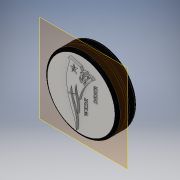
# Autodesk Inventor part: Wheel
Saved by Autodesk Inventor 2016 (Build 200138000, 138)
## iProperties
Created: 2016-10-07
Part Number: Wheel
Material: Generic
Document SubType Name: Modeling
Designer: desirw
Density: 1 g/cm^3
Appearance: Default
Mass: 52.9378 g
Surface Area: 147.304 cm^2
Volume: 52.9378 cm^3
Author: desirw
Autodesk Inventor part; units mm, degrees
ref_plane "YZ Plane" through (0, 0, 0) normal (1, 0, 0) x (0, 1, 0)
ref_plane "XZ Plane" through (0, 0, 0) normal (0, 1, 0) x (-1, 0, 0)
ref_plane "XY Plane" through (0, 0, 0) normal (0, 0, 1) x (1, 0, 0)
sketch "Sketch1" plane through (0, 0, 0) normal (0, 0, 1) x (1, 0, 0)
  circle A0 centre (0, 0) radius 31.75
  dimension "d0" = 63.5
  constraints: 1 centre point, 1 coincident
  measures "d0" diameter of A0
extrude "Extrusion1" add sketch "Sketch1" along normal blind 3.2512
sketch "Sketch2" plane through (0, 0, 3.2512) normal (0, 0, 1) x (1, 0, 0)
  circle A0 centre (0, 0) radius 33.655
  circle A1 centre (0, 0) radius 31.511
  circle A2 centre (0, 0) radius 31.511
  dimension "d3" = 67.31
  dimension "d40" = 2.144
  constraints: 3 centre point, 1 coincident
  measures "d3" diameter of A0
  measures "d40" radial gap between concentric circles of A1 A0
extrude "Extrusion2" add sketch "Sketch2" along normal blind 7.62 contours A0 | A1
sketch "Sketch3" plane through (0, 0, 0) normal (0, 0, -1) x (-1, 0, 0)
  circle A0 centre (0, 0) radius 33.655
  dimension "d6" = 67.31
  constraints: 1 centre point, 1 coincident
  measures "d6" diameter of A0
fillet "Fillet1" radius 2.54 1 edges at (-33.655, 0, 10.8712)
extrude "Extrusion3" add sketch "Sketch3" along normal blind 7.62
fillet "Fillet2" radius 2.54 1 edges at (33.655, 0, -7.62)
sketch "Sketch4" plane through (0, 0, -7.62) normal (0, 0, -1) x (-1, 0, 0)
  arc A0 (1.5256, -7.6067) -> (-1.5256, -7.6067) centre (0, -8.5367) ccw
  line L0 (1.5256, -7.6067) -> (10.0877, -14.0155)
  arc A1 (10.0877, -14.0155) -> (14.0155, -10.0877) centre (11.7691, -11.7691) ccw
  line L1 (14.0155, -10.0877) -> (7.6067, -1.5256)
  arc A2 (7.6067, 1.5256) -> (7.6067, -1.5256) centre (8.5367, 0) ccw
  line L2 (7.6067, 1.5256) -> (14.0155, 10.0877)
  arc A3 (14.0155, 10.0877) -> (10.0877, 14.0155) centre (11.7691, 11.7691) ccw
  line L3 (10.0877, 14.0155) -> (1.5256, 7.6067)
  arc A4 (-1.5256, 7.6067) -> (1.5256, 7.6067) centre (0, 8.5367) ccw
  line L4 (-1.5256, 7.6067) -> (-10.0877, 14.0155)
  arc A5 (-10.0877, 14.0155) -> (-14.0155, 10.0877) centre (-11.7691, 11.7691) ccw
  line L5 (-14.0155, 10.0877) -> (-7.6067, 1.5256)
  arc A6 (-7.6067, -1.5256) -> (-7.6067, 1.5256) centre (-8.5367, 0) ccw
  line L6 (-7.6067, -1.5256) -> (-14.0155, -10.0877)
  arc A7 (-14.0155, -10.0877) -> (-10.0877, -14.0155) centre (-11.7691, -11.7691) ccw
  line L7 (-10.0877, -14.0155) -> (-1.5256, -7.6067)
  circle A8 centre (12.339, -12.339) radius 0.75
  circle A9 centre (9.8641, -9.8641) radius 0.75
  circle A10 centre (7.3893, -7.3893) radius 0.75
  circle A11 centre (4.9144, -4.9144) radius 0.75
  circle A12 centre (12.339, 12.339) radius 0.75
  circle A13 centre (9.8641, 9.8641) radius 0.75
  circle A14 centre (7.3893, 7.3893) radius 0.75
  circle A15 centre (4.9144, 4.9144) radius 0.75
  circle A16 centre (-12.339, 12.339) radius 0.75
  circle A17 centre (-9.8641, 9.8641) radius 0.75
  circle A18 centre (-7.3893, 7.3893) radius 0.75
  circle A19 centre (-4.9144, 4.9144) radius 0.75
  circle A20 centre (-12.339, -12.339) radius 0.75
  circle A21 centre (-9.8641, -9.8641) radius 0.75
  circle A22 centre (-7.3893, -7.3893) radius 0.75
  circle A23 centre (-4.9144, -4.9144) radius 0.75
  circle A24 centre (0, 0) radius 3.6
  constraints: 25 centre point, 16 end point, 16 point on circle
extrude "Extrusion4" cut sketch "Sketch4" against normal blind 2.3622 contours A0 L7 A7 L6 A6 L5 A5 L4 A4 L3 A3 L2 A2 L1 A1 L0 | A8 | A9 | A10 | A11 | A12 | A13 | A14 | A15 | A16 | A17 | A18 | A19 | A20 | A21 | A22 | A23 | A24
sketch "Sketch5" plane through (0, 0, -7.62) normal (0, 0, -1) x (-1, 0, 0)
  circle A0 centre (0, 0) radius 3.6195
  dimension "d15" = 7.239
  constraints: 1 centre point, 1 coincident
  measures "d15" diameter of A0
extrude "Extrusion5" cut sketch "Sketch5" against normal blind 1.1684
sketch "Sketch6" plane through (0, 0, -5.2578) normal (0, 0, -1) x (-1, 0, 0)
  circle A0 centre (0, 0) radius 1.2446
  dimension "d16" = 2.4892
  constraints: 1 centre point, 1 coincident
  measures "d16" diameter of A0
extrude "Extrusion6" cut sketch "Sketch6" against normal blind 7.62
sketch "Sketch7" plane through (0, 0, 10.8712) normal (0, 0, 1) x (1, 0, 0)
  circle A0 centre (0, 0) radius 2.54
  dimension "d19" = 5.08
  constraints: 1 centre point, 1 coincident
  measures "d19" diameter of A0
extrude "Extrusion7" cut sketch "Sketch7" against normal blind 15.24
sketch "Sketch12" plane through (0, 0, -5.2578) normal (0, 0, -1) x (-1, 0, 0)
  circle A0 centre (0, 0) radius 3.5498
  circle A1 centre (0, 0) radius 3.6 projected
  dimension "d41" = 7.2
  constraints: 1 centre point, 1 coincident
  measures "d41" diameter of A1
extrude "Extrusion11" cut sketch "Sketch12" against normal blind 0.2286 contours A0
sketch "Sketch13" plane through (0, 0, -7.62) normal (0, 0, -1) x (-1, 0, 0)
  circle A0 centre (-9.8641, -9.8641) radius 1.0795
  circle A1 centre (-9.8641, 9.8641) radius 1.0795
  circle A2 centre (9.8641, 9.8641) radius 1.0795
  circle A3 centre (9.8641, -9.8641) radius 1.0795
  dimension "d46" = 2.159
  dimension "d48" = 2.159
  dimension "d49" = 2.159
  dimension "d50" = 2.159
  constraints: 4 centre point
  measures "d46" diameter of A0
  measures "d48" diameter of A2
  measures "d49" diameter of A3
  measures "d50" diameter of A1
extrude "Extrusion12" cut sketch "Sketch13" against normal blind 12.7
sketch "Sketch16" plane through (0, 0, 10.8712) normal (0, 0, 1) x (1, 0, 0)
  circle A0 centre (0, 0) radius 31.115 projected
  circle A1 centre (0, 0) radius 2.54 projected
  circle A2 centre (0, 0) radius 31.115
  constraints: 1 centre point, 1 coincident, 1 concentric
extrude "Extrusion13" cut sketch "Sketch16" against normal blind 2.54
sketch "Sketch17" plane through (0, 0, 8.3312) normal (0, 0, 1) x (1, 0, 0)
  circle A0 centre (0, 0) radius 1.2446 projected
  circle A1 centre (0, 0) radius 7.62
  circle A2 centre (0, 0) radius 29.21
  dimension "d56" = 15.24
  dimension "d60" = 58.42
  constraints: 2 centre point, 2 coincident
  measures "d56" diameter of A1
  measures "d60" diameter of A2
extrude "Extrusion14" cut sketch "Sketch17" against normal blind 12.7 contours A2
fillet "Fillet3" radius 3.175 2 edges at (-29.21, 0, 8.3312) (-7.62, 0, 8.3312)
sketch "Sketch20" plane through (0, 0, -7.62) normal (0, 0, -1) x (-1, 0, 0)
  circle A0 centre (19.0012, 0) radius 8.4433
  circle A1 centre (0, 0) radius 1.2446 projected
  circle A2 centre (0, 0) radius 2.54 projected
  circle A3 centre (0, -19.0012) radius 8.4433
  circle A4 centre (-19.0012, 0) radius 8.4433
  circle A5 centre (0, 19.0012) radius 8.4433
  arc A6 (15.9108, 14.6269) -> (13.5038, 17.0339) centre (16.1061, 17.2292) ccw construction
  arc A7 (15.8105, 13.2894) -> (12.1662, 16.9336) centre (16.1061, 17.2292) ccw
  arc A8 (16.0112, 15.9644) -> (14.8413, 17.1343) centre (16.1061, 17.2292) ccw
  arc A9 (16.0112, 15.9644) -> (15.8105, 13.2894) centre (15.9108, 14.6269) ccw
  arc A10 (12.1662, 16.9336) -> (14.8413, 17.1343) centre (13.5038, 17.0339) ccw
  arc A11 (14.6269, -15.9108) -> (17.0339, -13.5038) centre (17.2292, -16.1061) ccw construction
  arc A12 (13.2894, -15.8105) -> (16.9336, -12.1662) centre (17.2292, -16.1061) ccw
  arc A13 (15.9644, -16.0112) -> (17.1343, -14.8413) centre (17.2292, -16.1061) ccw
  arc A14 (15.9644, -16.0112) -> (13.2894, -15.8105) centre (14.6269, -15.9108) ccw
  arc A15 (16.9336, -12.1662) -> (17.1343, -14.8413) centre (17.0339, -13.5038) ccw
  arc A16 (-15.9108, -14.6269) -> (-13.5038, -17.0339) centre (-16.1061, -17.2292) ccw construction
  arc A17 (-15.8105, -13.2894) -> (-12.1662, -16.9336) centre (-16.1061, -17.2292) ccw
  arc A18 (-16.0112, -15.9644) -> (-14.8413, -17.1343) centre (-16.1061, -17.2292) ccw
  arc A19 (-16.0112, -15.9644) -> (-15.8105, -13.2894) centre (-15.9108, -14.6269) ccw
  arc A20 (-12.1662, -16.9336) -> (-14.8413, -17.1343) centre (-13.5038, -17.0339) ccw
  arc A21 (-14.6269, 15.9108) -> (-17.0339, 13.5038) centre (-17.2292, 16.1061) ccw construction
  arc A22 (-13.2894, 15.8105) -> (-16.9336, 12.1662) centre (-17.2292, 16.1061) ccw
  arc A23 (-15.9644, 16.0112) -> (-17.1343, 14.8413) centre (-17.2292, 16.1061) ccw
  arc A24 (-15.9644, 16.0112) -> (-13.2894, 15.8105) centre (-14.6269, 15.9108) ccw
  arc A25 (-16.9336, 12.1662) -> (-17.1343, 14.8413) centre (-17.0339, 13.5038) ccw
  dimension "d66" = 360
  dimension "d70" = 360
  constraints: 40 point on circle, 24 centre point, 4 coincident, 4 tangent, 67 other
extrude "Extrusion15" cut sketch "Sketch20" against normal blind 10.16 contours A0 | A3 | A4 | A5 | A9 A8 A10 A7 | A14 A13 A15 A12 | A19 A18 A20 A17 | A24 A23 A25 A22
sketch "Sketch21" plane through (0, 0, -4.3688) normal (0, 0, 1) x (1, 0, 0)
  circle A0 centre (-9.8653, -9.893) radius 2.159
  circle A1 centre (-9.8653, 9.8376) radius 2.159
  circle A2 centre (9.867, -9.893) radius 2.159
  circle A3 centre (9.867, 9.8376) radius 2.159
  point P0 (0, 0)
  dimension "d74" = 4.318
  dimension "d75" = 4.318
  dimension "d76" = 4.318
  dimension "d77" = 4.318
  constraints: 4 centre point
  measures "d74" diameter of A0
  measures "d75" diameter of A1
  measures "d76" diameter of A2
  measures "d77" diameter of A3
extrude "Extrusion16" cut sketch "Sketch21" against normal blind 0.254
sketch "Sketch23" plane through (0, 0, 8.3312) normal (0, 0, 1) x (1, 0, 0)
  circle A0 centre (0, 0) radius 8.0486
  constraints: 1 centre point, 1 coincident
extrude "Extrusion17" cut sketch "Sketch23" against normal blind 12.7
ref_plane "Work Plane2" through (0, 0, 8.3312) normal (0, 0, 1) x (1, 0, 0)
sketch "Sketch24" plane through (0, 0, 8.3312) normal (0, 0, 1) x (1, 0, 0)
  circle A0 centre (0, 0) radius 31.1534
  constraints: 1 centre point, 1 coincident
extrude "Extrusion18" add sketch "Sketch24" along normal blind 2.54
sketch "Sketch25" plane through (0, 0, 10.8712) normal (0, 0, 1) x (1, 0, 0)
  line L0 (-12.7986, -29.9392) -> (-12.7986, 28.2876) construction
  line L1 (-12.7986, 28.2876) -> (14.4515, 28.2876) construction
  line L2 (14.4515, 28.2876) -> (14.4515, -29.9392) construction
  line L3 (14.4515, -29.9392) -> (-12.7986, -29.9392) construction
  arc A0 (-2.4703, -28.2892) -> (-5.6682, -15.7345) centre (-39.8581, -31.1279) ccw
  arc A1 (-10.3026, -1.9948) -> (-5.6682, -15.7345) centre (146.9864, 43.407) ccw
  arc A2 (-2.4703, -28.2892) -> (-2.4703, -18.2629) centre (-33.8456, -23.2761) ccw
  arc A3 (-2.4703, -18.2629) -> (-5.2168, -8.4433) centre (-79.7357, -34.5801) ccw
  arc A4 (-7.0459, -1.252) -> (-5.2168, -8.4433) centre (32.2007, 4.9019) ccw
  line L4 (-10.3026, -1.9948) -> (-7.0459, -1.252)
  arc A5 (-1.4091, -14.8666) -> (-3.8781, -5.8135) centre (-42.9348, -21.3286) ccw
  arc A6 (-5.6682, -0.6984) -> (-3.8781, -5.8135) centre (38.7717, 11.9828) ccw
  arc A7 (-2.9605, 0) -> (-5.6682, -0.6984) centre (0.5008, -19.0171) ccw
  arc A8 (-1.7257, -5.5998) -> (-2.9605, 0) centre (-46.1597, -12.462) ccw
  arc A9 (-1.4091, -14.8666) -> (-1.7257, -5.5998) centre (-31.0492, -11.2405) ccw
  arc A10 (13.0542, 18.6707) -> (0.223, -3.0699) centre (34.2938, -8.5214) ccw
  arc A11 (13.0542, 18.6707) -> (11.4718, 20.2531) centre (10.1474, 17.3464) ccw
  arc A12 (11.4718, 20.2531) -> (9.4266, 20.0581) centre (10.5991, 18.5838) ccw
  arc A13 (9.4266, 20.0581) -> (8.2975, 20.459) centre (7.7468, 17.1172) ccw
  arc A14 (8.2975, 20.459) -> (7.2209, 20.5419) centre (7.4283, 16.2053) ccw
  arc A15 (6.4262, 22.0118) -> (7.2209, 20.5419) centre (11.9084, 24.0263) ccw
  arc A16 (2.6562, 21.2483) -> (6.4262, 22.0118) centre (-20.9306, 147.4079) ccw
  arc A17 (2.6562, 21.2483) -> (1.1935, 24.0263) centre (-252.5291, -111.3406) ccw
  arc A18 (1.1935, 24.0263) -> (-9.4849, 27.0616) centre (-900.7825, -3128.8756) ccw
  arc A19 (-9.1238, 22.0118) -> (-9.4849, 27.0616) centre (-21.4008, 23.6716) ccw
  arc A20 (-10.3026, 17.8312) -> (-9.1238, 22.0118) centre (-36.152, 27.3765) ccw
  arc A21 (-10.3026, 17.8312) -> (-11.3285, 12.6153) centre (170.6673, -20.4736) ccw
  arc A22 (-11.3285, 12.6153) -> (-10.3026, -1.252) centre (38.6762, 9.3432) ccw
  arc A23 (-7.374, -0.5894) -> (-10.3026, -1.252) centre (0.434, -41.9034) ccw
  arc A24 (-6.6405, 5.393) -> (-7.374, -0.5894) centre (2.9307, 1.1832) ccw
  arc A25 (-6.6405, 5.393) -> (-5.8275, -0.1263) centre (42.4689, 9.8072) ccw
  arc A26 (-3.1357, 0.5919) -> (-5.8275, -0.1263) centre (0.6817, -19.118) ccw
  arc A27 (-2.2091, 8.7203) -> (-3.1357, 0.5919) centre (7.8506, 3.4565) ccw
  arc A28 (-2.2091, 8.7203) -> (-1.4091, 2.4558) centre (41.2883, 11.0914) ccw
  arc A29 (0.223, -3.0699) -> (-1.4091, 2.4558) centre (-65.3016, -19.4203) ccw
  arc A30 (6.7707, 15.7398) -> (4.847, 15.3673) centre (16.1173, -37.684) ccw
  arc A31 (4.847, 15.3673) -> (2.5284, 11.9828) centre (51.1574, -18.8455) ccw
  arc A32 (2.0647, 12.0311) -> (2.5284, 11.9828) centre (2.3182, 12.2154) ccw
  arc A33 (0.6817, 14.3084) -> (2.0647, 12.0311) centre (3.8781, 14.6909) ccw
  arc A34 (1.0059, 16.9464) -> (0.6817, 14.3084) centre (8.9448, 14.6319) ccw
  arc A35 (1.507, 17.4809) -> (1.0059, 16.9464) centre (1.5569, 16.9319) ccw
  arc A36 (1.507, 17.4809) -> (1.791, 15.7398) centre (3.5637, 16.9227) ccw
  arc A37 (1.791, 15.7398) -> (2.9878, 14.8708) centre (3.5637, 16.9227) ccw
  line L5 (2.9878, 14.8708) -> (2.9878, 18.3662)
  arc A38 (1.4604, 19.4854) -> (2.9878, 18.3662) centre (3.1078, 20.1318) ccw
  arc A39 (1.3568, 19.6561) -> (1.4604, 19.4854) centre (1.5862, 19.6786) ccw
  arc A40 (1.3568, 20.1992) -> (1.3568, 19.6561) centre (2.2724, 19.9277) ccw
  arc A41 (5.9606, 21.1505) -> (1.3568, 20.1992) centre (8.9783, -5.0691) ccw
  line L6 (5.9606, 21.1505) -> (5.9606, 18.988)
  arc A42 (5.9606, 18.988) -> (6.2957, 18.7748) centre (9.575, 24.2979) ccw
  arc A43 (6.2957, 18.7748) -> (6.9567, 19.9277) centre (-103.158, 82.2966) ccw
  arc A44 (7.5209, 19.9277) -> (6.9567, 19.9277) centre (7.2388, 19.3131) ccw
  line L7 (7.5209, 19.9277) -> (7.5209, 18.6986)
  arc A45 (8.344, 17.7097) -> (7.5209, 18.6986) centre (6.084, 16.6658) ccw
  arc A46 (8.344, 17.7097) -> (8.1842, 18.8788) centre (6.4633, 18.0481) ccw
  line L8 (8.1842, 18.8788) -> (8.1842, 20.0692)
  line L9 (8.1842, 20.0692) -> (8.4773, 20.0692)
  arc A47 (9.1501, 19.6561) -> (8.4773, 20.0692) centre (8.1291, 18.7477) ccw
  line L10 (9.1501, 19.6561) -> (9.1501, 18.878)
  arc A48 (10.3252, 19.7825) -> (9.1501, 18.878) centre (11.157, 17.4862) ccw
  line L11 (10.3252, 19.7825) -> (10.9883, 19.7825)
  arc A49 (12.0805, 18.8788) -> (10.9883, 19.7825) centre (10.1284, 17.6314) ccw
  arc A50 (12.0805, 18.8788) -> (5.0259, 10.9955) centre (36.9587, -10.4824) ccw
  arc A51 (4.3066, 11.9036) -> (5.0259, 10.9955) centre (5.7027, 12.2705) ccw
  arc A52 (4.3066, 12.6373) -> (4.3066, 11.9036) centre (5.7027, 12.2705) ccw
  arc A53 (6.7707, 15.7398) -> (4.3066, 12.6373) centre (9.0478, 11.4015) ccw
  line L12 (-3.2282, 19.8186) -> (-2.0723, 16.5796)
  line L13 (-2.0723, 16.5796) -> (-4.5876, 18.4941)
  line L14 (-4.5876, 18.4941) -> (-6.5126, 16.6185)
  line L15 (-6.5126, 16.6185) -> (-5.8751, 19.474)
  line L16 (-5.8751, 19.474) -> (-7.5613, 20.8788)
  line L17 (-7.5613, 20.8788) -> (-5.366, 21.4271)
  line L18 (-5.366, 21.4271) -> (-4.6252, 24.0672)
  line L19 (-4.6252, 24.0672) -> (-3.8073, 21.7551)
  line L20 (-3.8073, 21.7551) -> (-0.8504, 22.1353)
  line L21 (-0.8504, 22.1353) -> (-3.2282, 19.8186)
  point P0 (0, 0)
  constraints: 110 point on circle, 54 centre point, 36 end point, 5 vertical, 3 concentric, 2 point on line, 1 collinear, 1 horizontal, 1 perpendicular, 2 other
extrude "Extrusion19" add sketch "Sketch25" along normal blind 2.032
sketch "Sketch26" plane through (0, 0, 10.8712) normal (0, 0, 1) x (1, 0, 0)
  line L0 (3.1838, -14.6945) -> (3.1838, -9.0616) construction
  line L1 (3.1838, -9.0616) -> (14.0414, -9.0616) construction
  line L2 (14.0414, -9.0616) -> (14.0414, -14.6945) construction
  line L3 (14.0414, -14.6945) -> (3.1838, -14.6945) construction
  line L4 (11.7993, -0.1306) -> (11.8156, 13.1695) construction
  line L5 (11.8156, 13.1695) -> (15.003, 13.1656) construction
  line L6 (15.003, 13.1656) -> (14.9868, -0.1345) construction
  line L7 (14.9868, -0.1345) -> (11.7993, -0.1306) construction
  line L8 (3.1838, -9.945) -> (3.2694, -9.945)
  spline S0 degree 2 poles (3.2694, -9.945) (3.2772, -10.0332) (3.3602, -10.1551) (3.4484, -10.2018) knots 0 0 0 1 2 2 2
  spline S1 degree 2 poles (3.4484, -10.2018) (3.4769, -10.2148) (3.8116, -10.3471) knots 0 0 0 1 1 1
  line L9 (3.8116, -10.3471) -> (6.4314, -11.3431)
  line L10 (6.4314, -11.3431) -> (6.4314, -11.4339)
  line L11 (6.4314, -11.4339) -> (4.3744, -12.2199)
  line L12 (4.3744, -12.2199) -> (6.4314, -13.0863)
  line L13 (6.4314, -13.0863) -> (6.4314, -13.1719)
  line L14 (6.4314, -13.1719) -> (3.8375, -14.2172)
  spline S2 degree 2 poles (3.8375, -14.2172) (3.4484, -14.3755) (3.2824, -14.5026) (3.2694, -14.653) knots 0 0 0 1 2 2 2
  line L15 (3.2694, -14.653) -> (3.1838, -14.653)
  line L16 (3.1838, -14.653) -> (3.1838, -13.2782)
  line L17 (3.1838, -13.2782) -> (3.2694, -13.2782)
  spline S3 degree 2 poles (3.2694, -13.2782) (3.2746, -13.4442) (3.3654, -13.5532) (3.4328, -13.5532) knots 0 0 0 1 2 2 2
  spline S4 degree 2 poles (3.4328, -13.5532) (3.5236, -13.5532) (3.8116, -13.4391) knots 0 0 0 1 1 1
  line L18 (3.8116, -13.4391) -> (5.3524, -12.8165)
  line L19 (5.3524, -12.8165) -> (4.1462, -12.3159)
  line L20 (4.1462, -12.3159) -> (3.8116, -12.4456)
  spline S5 degree 2 poles (3.8116, -12.4456) (3.534, -12.5545) (3.3498, -12.6712) (3.2694, -12.8217) (3.2694, -12.9696) knots 0 0 0 1 2 3 3 3
  line L21 (3.2694, -12.9696) -> (3.1838, -12.9696)
  line L22 (3.1838, -12.9696) -> (3.1838, -11.4339)
  line L23 (3.1838, -11.4339) -> (3.2694, -11.4339)
  spline S6 degree 2 poles (3.2694, -11.4339) (3.272, -11.5974) (3.2954, -11.6674) knots 0 0 0 1 1 1
  spline S7 degree 2 poles (3.2954, -11.6674) (3.3109, -11.7167) (3.3887, -11.7711) (3.438, -11.7711) knots 0 0 0 1 2 2 2
  spline S8 degree 2 poles (3.438, -11.7711) (3.4925, -11.7711) (3.77, -11.6674) knots 0 0 0 1 1 1
  line L24 (3.77, -11.6674) -> (5.2719, -11.0889)
  line L25 (5.2719, -11.0889) -> (3.9127, -10.5701)
  spline S9 degree 2 poles (3.9127, -10.5701) (3.7, -10.4897) (3.547, -10.4508) (3.4795, -10.4508) knots 0 0 0 1 2 2 2
  spline S10 degree 2 poles (3.4795, -10.4508) (3.3835, -10.4508) (3.2746, -10.5831) (3.2694, -10.7673) knots 0 0 0 1 2 2 2
  line L26 (3.2694, -10.7673) -> (3.1838, -10.7673)
  line L27 (3.1838, -10.7673) -> (3.1838, -9.945)
  line L28 (3.3654, -8.5936) -> (4.6572, -8.5936)
  line L29 (4.6572, -8.5936) -> (4.6572, -8.5287)
  spline S11 degree 2 poles (4.6572, -8.5287) (4.6572, -8.2252) (4.2785, -7.9528) (3.9075, -7.9139) knots 0 0 0 1 2 2 2
  line L30 (3.9075, -7.9139) -> (3.9075, -7.8283)
  line L31 (3.9075, -7.8283) -> (5.5703, -7.8283)
  line L32 (5.5703, -7.8283) -> (5.5703, -7.9139)
  spline S12 degree 2 poles (5.5703, -7.9139) (5.2979, -7.9425) (4.9529, -8.124) (4.8336, -8.3653) (4.8336, -8.5936) knots 0 0 0 1 2 3 3 3
  line L33 (4.8336, -8.5936) -> (5.7285, -8.5936)
  spline S13 degree 2 poles (5.7285, -8.5936) (5.9905, -8.5936) (6.1072, -8.5495) (6.1824, -8.4275) (6.1824, -8.2901) knots 0 0 0 1 2 3 3 3
  line L34 (6.1824, -8.2901) -> (6.1824, -8.1007)
  spline S14 degree 2 poles (6.1824, -8.1007) (6.1824, -7.6545) (5.77, -7.1176) (5.3498, -7.0009) knots 0 0 0 1 2 2 2
  line L35 (5.3498, -7.0009) -> (5.3498, -6.9153)
  line L36 (5.3498, -6.9153) -> (6.3588, -7.0579)
  line L37 (6.3588, -7.0579) -> (6.3588, -9.8023)
  line L38 (6.3588, -9.8023) -> (6.2732, -9.8023)
  line L39 (6.2732, -9.8023) -> (6.2732, -9.696)
  spline S15 degree 2 poles (6.2732, -9.696) (6.2732, -9.5585) (6.2239, -9.4755) knots 0 0 0 1 1 1
  spline S16 degree 2 poles (6.2239, -9.4755) (6.1902, -9.4158) (6.1124, -9.3821) knots 0 0 0 1 1 1
  spline S17 degree 2 poles (6.1124, -9.3821) (6.0553, -9.3562) (5.8167, -9.3562) knots 0 0 0 1 1 1
  line L40 (5.8167, -9.3562) -> (3.726, -9.3562)
  spline S18 degree 2 poles (3.726, -9.3562) (3.5107, -9.3562) (3.4614, -9.3665) knots 0 0 0 1 1 1
  spline S19 degree 2 poles (3.4614, -9.3665) (3.3784, -9.3925) (3.3343, -9.4547) knots 0 0 0 1 1 1
  spline S20 degree 2 poles (3.3343, -9.4547) (3.2694, -9.5429) (3.2694, -9.696) knots 0 0 0 1 1 1
  line L41 (3.2694, -9.696) -> (3.2694, -9.8023)
  line L42 (3.2694, -9.8023) -> (3.1838, -9.8023)
  line L43 (3.1838, -9.8023) -> (3.1838, -7.1435)
  line L44 (3.1838, -7.1435) -> (4.1228, -7.1435)
  line L45 (4.1228, -7.1435) -> (4.1228, -7.2291)
  spline S21 degree 2 poles (4.1228, -7.2291) (3.7778, -7.2966) (3.4769, -7.5456) (3.4069, -7.7713) knots 0 0 0 1 2 2 2
  spline S22 degree 2 poles (3.4069, -7.7713) (3.3654, -7.901) (3.3654, -8.2641) knots 0 0 0 1 1 1
  line L46 (3.3654, -8.2641) -> (3.3654, -8.5936)
  line L47 (6.3588, -6.6351) -> (6.2732, -6.6351)
  line L48 (6.2732, -6.6351) -> (6.2732, -6.5288)
  spline S23 degree 2 poles (6.2732, -6.5288) (6.2732, -6.3913) (6.1876, -6.246) (6.1124, -6.2097) knots 0 0 0 1 2 2 2
  spline S24 degree 2 poles (6.1124, -6.2097) (6.0631, -6.189) (5.8167, -6.189) knots 0 0 0 1 1 1
  line L49 (5.8167, -6.189) -> (3.726, -6.189)
  spline S25 degree 2 poles (3.726, -6.189) (3.4821, -6.189) (3.3602, -6.2408) (3.2694, -6.3965) (3.2694, -6.5288) knots 0 0 0 1 2 3 3 3
  line L50 (3.2694, -6.5288) -> (3.2694, -6.6351)
  line L51 (3.2694, -6.6351) -> (3.1838, -6.6351)
  line L52 (3.1838, -6.6351) -> (3.1838, -5.2162)
  spline S26 degree 2 poles (3.1838, -5.2162) (3.1838, -4.6456) (3.3395, -4.3006) knots 0 0 0 1 1 1
  spline S27 degree 2 poles (3.3395, -4.3006) (3.5288, -3.8777) (4.2966, -3.4394) (4.7817, -3.4394) knots 0 0 0 1 2 2 2
  spline S28 degree 2 poles (4.7817, -3.4394) (5.1163, -3.4394) (5.6792, -3.6547) (6.0475, -3.9971) (6.2706, -4.4432) (6.3303, -4.7649) knots 0 0 0 1 2 3 4 4 4
  spline S29 degree 2 poles (6.3303, -4.7649) (6.3588, -4.9075) (6.3588, -5.2162) knots 0 0 0 1 1 1
  line L53 (6.3588, -5.2162) -> (6.3588, -6.6351)
  line L54 (3.3654, -5.4263) -> (5.84, -5.4263)
  spline S30 degree 2 poles (5.84, -5.4263) (6.0346, -5.4263) (6.1228, -5.39) (6.1461, -5.3433) knots 0 0 0 1 2 2 2
  spline S31 degree 2 poles (6.1461, -5.3433) (6.1824, -5.2811) (6.1824, -5.1618) knots 0 0 0 1 1 1
  spline S32 degree 2 poles (6.1824, -5.1618) (6.1824, -4.7727) (5.9152, -4.5651) knots 0 0 0 1 1 1
  spline S33 degree 2 poles (5.9152, -4.5651) (5.5547, -4.285) (4.7973, -4.285) knots 0 0 0 1 1 1
  spline S34 degree 2 poles (4.7973, -4.285) (4.1877, -4.285) (3.8245, -4.4769) knots 0 0 0 1 1 1
  spline S35 degree 2 poles (3.8245, -4.4769) (3.5392, -4.63) (3.4354, -4.8686) knots 0 0 0 1 1 1
  spline S36 degree 2 poles (3.4354, -4.8686) (3.3628, -5.0346) (3.3654, -5.4263) knots 0 0 0 1 1 1
  line L55 (3.3654, -1.9323) -> (4.6572, -1.9323)
  line L56 (4.6572, -1.9323) -> (4.6572, -1.8674)
  spline S37 degree 2 poles (4.6572, -1.8674) (4.6572, -1.5639) (4.2785, -1.2916) (3.9075, -1.2527) knots 0 0 0 1 2 2 2
  line L57 (3.9075, -1.2527) -> (3.9075, -1.1671)
  line L58 (3.9075, -1.1671) -> (5.5703, -1.1671)
  line L59 (5.5703, -1.1671) -> (5.5703, -1.2527)
  spline S38 degree 2 poles (5.5703, -1.2527) (5.2979, -1.2812) (4.9529, -1.4628) (4.8336, -1.704) (4.8336, -1.9323) knots 0 0 0 1 2 3 3 3
  line L60 (4.8336, -1.9323) -> (5.7285, -1.9323)
  spline S39 degree 2 poles (5.7285, -1.9323) (5.9905, -1.9323) (6.1072, -1.8882) (6.1824, -1.7663) (6.1824, -1.6288) knots 0 0 0 1 2 3 3 3
  line L61 (6.1824, -1.6288) -> (6.1824, -1.4394)
  spline S40 degree 2 poles (6.1824, -1.4394) (6.1824, -0.9933) (5.77, -0.4563) (5.3498, -0.3396) knots 0 0 0 1 2 2 2
  line L62 (5.3498, -0.3396) -> (5.3498, -0.254)
  line L63 (5.3498, -0.254) -> (6.3588, -0.3967)
  line L64 (6.3588, -0.3967) -> (6.3588, -3.1411)
  line L65 (6.3588, -3.1411) -> (6.2732, -3.1411)
  line L66 (6.2732, -3.1411) -> (6.2732, -3.0347)
  spline S41 degree 2 poles (6.2732, -3.0347) (6.2732, -2.8972) (6.2239, -2.8142) knots 0 0 0 1 1 1
  spline S42 degree 2 poles (6.2239, -2.8142) (6.1902, -2.7546) (6.1124, -2.7208) knots 0 0 0 1 1 1
  spline S43 degree 2 poles (6.1124, -2.7208) (6.0553, -2.6949) (5.8167, -2.6949) knots 0 0 0 1 1 1
  line L67 (5.8167, -2.6949) -> (3.726, -2.6949)
  spline S44 degree 2 poles (3.726, -2.6949) (3.5107, -2.6949) (3.4614, -2.7053) knots 0 0 0 1 1 1
  spline S45 degree 2 poles (3.4614, -2.7053) (3.3784, -2.7312) (3.3343, -2.7935) knots 0 0 0 1 1 1
  spline S46 degree 2 poles (3.3343, -2.7935) (3.2694, -2.8817) (3.2694, -3.0347) knots 0 0 0 1 1 1
  line L68 (3.2694, -3.0347) -> (3.2694, -3.1411)
  line L69 (3.2694, -3.1411) -> (3.1838, -3.1411)
  line L70 (3.1838, -3.1411) -> (3.1838, -0.4823)
  line L71 (3.1838, -0.4823) -> (4.1228, -0.4823)
  line L72 (4.1228, -0.4823) -> (4.1228, -0.5679)
  spline S47 degree 2 poles (4.1228, -0.5679) (3.7778, -0.6353) (3.4769, -0.8843) (3.4069, -1.11) knots 0 0 0 1 2 2 2
  spline S48 degree 2 poles (3.4069, -1.11) (3.3654, -1.2397) (3.3654, -1.6028) knots 0 0 0 1 1 1
  line L73 (3.3654, -1.6028) -> (3.3654, -1.9323)
  line L74 (14.9171, -0.0722) -> (14.835, -0.0721)
  line L75 (14.835, -0.0721) -> (14.8351, 0.03)
  spline S49 degree 2 poles (14.8351, 0.03) (14.8352, 0.162) (14.7532, 0.3016) (14.6811, 0.3365) knots 0 0 0 1 2 2 2
  spline S50 degree 2 poles (14.6811, 0.3365) (14.6338, 0.3565) (14.3972, 0.3568) knots 0 0 0 1 1 1
  line L76 (14.3972, 0.3568) -> (12.3901, 0.3592)
  spline S51 degree 2 poles (12.3901, 0.3592) (12.156, 0.3595) (12.0389, 0.3099) (11.9516, 0.1606) (11.9514, 0.0336) knots 0 0 0 1 2 3 3 3
  line L77 (11.9514, 0.0336) -> (11.9513, -0.0685)
  line L78 (11.9513, -0.0685) -> (11.8691, -0.0684)
  line L79 (11.8691, -0.0684) -> (11.8708, 1.2937)
  spline S52 degree 2 poles (11.8708, 1.2937) (11.8715, 1.8415) (12.0213, 2.1726) knots 0 0 0 1 1 1
  spline S53 degree 2 poles (12.0213, 2.1726) (12.2036, 2.5782) (12.9412, 2.9982) (13.4069, 2.9976) knots 0 0 0 1 2 2 2
  spline S54 degree 2 poles (13.4069, 2.9976) (13.7281, 2.9972) (14.2682, 2.7899) (14.6214, 2.4607) (14.835, 2.0322) (14.8919, 1.7233) knots 0 0 0 1 2 3 4 4 4
  spline S55 degree 2 poles (14.8919, 1.7233) (14.9192, 1.5863) (14.9188, 1.29) knots 0 0 0 1 1 1
  line L80 (14.9188, 1.29) -> (14.9171, -0.0722)
  line L81 (12.0449, 1.0918) -> (14.4205, 1.0889)
  spline S56 degree 2 poles (14.4205, 1.0889) (14.6073, 1.0887) (14.692, 1.1234) (14.7145, 1.1682) knots 0 0 0 1 2 2 2
  spline S57 degree 2 poles (14.7145, 1.1682) (14.7494, 1.2279) (14.7495, 1.3425) knots 0 0 0 1 1 1
  spline S58 degree 2 poles (14.7495, 1.3425) (14.75, 1.716) (14.4937, 1.9155) knots 0 0 0 1 1 1
  spline S59 degree 2 poles (14.4937, 1.9155) (14.1479, 2.1849) (13.4208, 2.1858) knots 0 0 0 1 1 1
  spline S60 degree 2 poles (13.4208, 2.1858) (12.8356, 2.1865) (12.4868, 2.0027) knots 0 0 0 1 1 1
  spline S61 degree 2 poles (12.4868, 2.0027) (12.2127, 1.8561) (12.1128, 1.6271) knots 0 0 0 1 1 1
  spline S62 degree 2 poles (12.1128, 1.6271) (12.0428, 1.4678) (12.0449, 1.0918) knots 0 0 0 1 1 1
  line L82 (12.049, 4.4461) -> (13.2891, 4.4446)
  line L83 (13.2891, 4.4446) -> (13.2892, 4.5068)
  spline S63 degree 2 poles (13.2892, 4.5068) (13.2895, 4.7982) (12.9263, 5.0601) (12.5702, 5.0979) knots 0 0 0 1 2 2 2
  line L84 (12.5702, 5.0979) -> (12.5703, 5.18)
  line L85 (12.5703, 5.18) -> (14.1665, 5.1781)
  line L86 (14.1665, 5.1781) -> (14.1664, 5.0959)
  spline S64 degree 2 poles (14.1664, 5.0959) (13.9049, 5.0688) (13.5735, 4.8949) (13.4587, 4.6635) (13.4584, 4.4444) knots 0 0 0 1 2 3 3 3
  line L87 (13.4584, 4.4444) -> (14.3175, 4.4433)
  spline S65 degree 2 poles (14.3175, 4.4433) (14.569, 4.443) (14.6812, 4.4852) (14.7535, 4.6021) (14.7537, 4.7341) knots 0 0 0 1 2 3 3 3
  line L88 (14.7537, 4.7341) -> (14.7539, 4.9159)
  spline S66 degree 2 poles (14.7539, 4.9159) (14.7544, 5.3442) (14.3591, 5.8602) (13.9558, 5.9727) knots 0 0 0 1 2 2 2
  line L89 (13.9558, 5.9727) -> (13.9559, 6.0549)
  line L90 (13.9559, 6.0549) -> (14.9245, 5.9168)
  line L91 (14.9245, 5.9168) -> (14.9212, 3.2821)
  line L92 (14.9212, 3.2821) -> (14.8391, 3.2822)
  line L93 (14.8391, 3.2822) -> (14.8392, 3.3843)
  spline S67 degree 2 poles (14.8392, 3.3843) (14.8393, 3.5163) (14.7921, 3.5961) knots 0 0 0 1 1 1
  spline S68 degree 2 poles (14.7921, 3.5961) (14.7598, 3.6534) (14.6852, 3.6858) knots 0 0 0 1 1 1
  spline S69 degree 2 poles (14.6852, 3.6858) (14.6304, 3.7108) (14.4013, 3.7111) knots 0 0 0 1 1 1
  line L94 (14.4013, 3.7111) -> (12.3942, 3.7135)
  spline S70 degree 2 poles (12.3942, 3.7135) (12.1875, 3.7138) (12.1402, 3.7039) knots 0 0 0 1 1 1
  spline S71 degree 2 poles (12.1402, 3.7039) (12.0605, 3.6791) (12.0181, 3.6194) knots 0 0 0 1 1 1
  spline S72 degree 2 poles (12.0181, 3.6194) (11.9557, 3.5348) (11.9555, 3.3879) knots 0 0 0 1 1 1
  line L95 (11.9555, 3.3879) -> (11.9554, 3.2858)
  line L96 (11.9554, 3.2858) -> (11.8732, 3.2859)
  line L97 (11.8732, 3.2859) -> (11.8764, 5.8383)
  line L98 (11.8764, 5.8383) -> (12.7778, 5.8372)
  line L99 (12.7778, 5.8372) -> (12.7777, 5.755)
  spline S73 degree 2 poles (12.7777, 5.755) (12.4464, 5.6907) (12.1573, 5.452) (12.0898, 5.2354) knots 0 0 0 1 2 2 2
  spline S74 degree 2 poles (12.0898, 5.2354) (12.0498, 5.111) (12.0494, 4.7623) knots 0 0 0 1 1 1
  line L100 (12.0494, 4.7623) -> (12.049, 4.4461)
  line L101 (11.8098, 8.4257) -> (12.8258, 8.4494)
  line L102 (12.8258, 8.4494) -> (12.8257, 8.3572)
  spline S75 degree 2 poles (12.8257, 8.3572) (12.4446, 8.2929) (11.9783, 7.7805) (11.978, 7.4842) knots 0 0 0 1 2 2 2
  spline S76 degree 2 poles (11.978, 7.4842) (11.9777, 7.2551) (12.2214, 6.9859) (12.3808, 6.9857) knots 0 0 0 1 2 2 2
  spline S77 degree 2 poles (12.3808, 6.9857) (12.4829, 6.9855) (12.5601, 7.0328) knots 0 0 0 1 1 1
  spline S78 degree 2 poles (12.5601, 7.0328) (12.6673, 7.0974) (12.7696, 7.2417) knots 0 0 0 1 1 1
  spline S79 degree 2 poles (12.7696, 7.2417) (12.8444, 7.3487) (13.0341, 7.7319) knots 0 0 0 1 1 1
  spline S80 degree 2 poles (13.0341, 7.7319) (13.2962, 8.267) (13.5306, 8.4535) knots 0 0 0 1 1 1
  spline S81 degree 2 poles (13.5306, 8.4535) (13.7649, 8.6375) (14.0662, 8.6371) knots 0 0 0 1 1 1
  spline S82 degree 2 poles (14.0662, 8.6371) (14.4472, 8.6366) (14.9968, 8.0408) (14.9962, 7.5801) knots 0 0 0 1 2 2 2
  spline S83 degree 2 poles (14.9962, 7.5801) (14.996, 7.4357) (14.9385, 7.1793) (14.856, 6.9876) knots 0 0 0 1 2 2 2
  spline S84 degree 2 poles (14.856, 6.9876) (14.8111, 6.8781) (14.811, 6.8084) knots 0 0 0 1 1 1
  spline S85 degree 2 poles (14.811, 6.8084) (14.8109, 6.7511) (14.9029, 6.619) (14.995, 6.5791) knots 0 0 0 1 2 2 2
  line L103 (14.995, 6.5791) -> (14.9949, 6.4969)
  line L104 (14.9949, 6.4969) -> (13.8444, 6.4983)
  line L105 (13.8444, 6.4983) -> (13.8445, 6.5805)
  spline S86 degree 2 poles (13.8445, 6.5805) (14.3302, 6.6795) (14.8389, 7.2441) (14.8393, 7.5704) knots 0 0 0 1 2 2 2
  spline S87 degree 2 poles (14.8393, 7.5704) (14.8396, 7.8219) (14.5661, 8.121) (14.3843, 8.1212) knots 0 0 0 1 2 2 2
  spline S88 degree 2 poles (14.3843, 8.1212) (14.2772, 8.1214) (14.0729, 8.0071) (13.8908, 7.7732) (13.746, 7.4746) knots 0 0 0 1 2 3 3 3
  spline S89 degree 2 poles (13.746, 7.4746) (13.5413, 7.059) (13.252, 6.6957) (12.8982, 6.5019) (12.684, 6.5022) knots 0 0 0 1 2 3 3 3
  spline S90 degree 2 poles (12.684, 6.5022) (12.3204, 6.5026) (11.8081, 7.0387) (11.8086, 7.4446) knots 0 0 0 1 2 2 2
  spline S91 degree 2 poles (11.8086, 7.4446) (11.8088, 7.594) (11.8438, 7.7334) knots 0 0 0 1 1 1
  spline S92 degree 2 poles (11.8438, 7.7334) (11.8713, 7.8379) (12.0186, 8.1416) (12.0187, 8.2038) knots 0 0 0 1 2 2 2
  spline S93 degree 2 poles (12.0187, 8.2038) (12.0188, 8.2611) (11.9466, 8.3284) (11.8097, 8.3585) knots 0 0 0 1 2 2 2
  line L106 (11.8097, 8.3585) -> (11.8098, 8.4257)
  line L107 (14.8479, 10.5013) -> (14.9301, 10.5012)
  line L108 (14.9301, 10.5012) -> (14.9281, 8.9125)
  line L109 (14.9281, 8.9125) -> (14.8459, 8.9126)
  line L110 (14.8459, 8.9126) -> (14.8461, 9.0147)
  spline S94 degree 2 poles (14.8461, 9.0147) (14.8462, 9.1466) (14.799, 9.2264) knots 0 0 0 1 1 1
  spline S95 degree 2 poles (14.799, 9.2264) (14.7667, 9.2837) (14.692, 9.3162) knots 0 0 0 1 1 1
  spline S96 degree 2 poles (14.692, 9.3162) (14.6373, 9.3411) (14.4082, 9.3414) knots 0 0 0 1 1 1
  line L111 (14.4082, 9.3414) -> (12.4011, 9.3439)
  spline S97 degree 2 poles (12.4011, 9.3439) (12.167, 9.3441) (12.0499, 9.2945) (11.9626, 9.1452) (11.9624, 9.0182) knots 0 0 0 1 2 3 3 3
  line L112 (11.9624, 9.0182) -> (11.9623, 8.9161)
  line L113 (11.9623, 8.9161) -> (11.8801, 8.9162)
  line L114 (11.8801, 8.9162) -> (11.8821, 10.5049)
  line L115 (11.8821, 10.5049) -> (11.9642, 10.5048)
  line L116 (11.9642, 10.5048) -> (11.9641, 10.4052)
  spline S98 degree 2 poles (11.9641, 10.4052) (11.964, 10.2732) (12.0112, 10.1935) knots 0 0 0 1 1 1
  spline S99 degree 2 poles (12.0112, 10.1935) (12.0435, 10.1337) (12.1181, 10.1012) knots 0 0 0 1 1 1
  spline S100 degree 2 poles (12.1181, 10.1012) (12.1729, 10.0763) (12.402, 10.076) knots 0 0 0 1 1 1
  line L117 (12.402, 10.076) -> (14.4091, 10.0735)
  spline S101 degree 2 poles (14.4091, 10.0735) (14.6432, 10.0732) (14.7603, 10.1254) (14.8476, 10.2747) (14.8478, 10.4017) knots 0 0 0 1 2 3 3 3
  line L118 (14.8478, 10.4017) -> (14.8479, 10.5013)
  line L119 (13.5422, 11.8376) -> (14.3963, 11.8366)
  spline S102 degree 2 poles (14.3963, 11.8366) (14.6453, 11.8363) (14.7724, 11.8959) (14.8498, 12.0502) (14.85, 12.2594) knots 0 0 0 1 2 3 3 3
  line L120 (14.85, 12.2594) -> (14.9322, 12.2593)
  line L121 (14.9322, 12.2593) -> (14.9303, 10.6979)
  line L122 (14.9303, 10.6979) -> (14.8481, 10.698)
  spline S103 degree 2 poles (14.8481, 10.698) (14.8484, 10.9097) (14.7689, 11.0617) (14.6444, 11.1216) (14.3954, 11.1219) knots 0 0 0 1 2 3 3 3
  line L123 (14.3954, 11.1219) -> (12.4182, 11.1243)
  spline S104 degree 2 poles (12.4182, 11.1243) (12.1692, 11.1246) (12.0421, 11.065) (11.9647, 10.9107) (11.9645, 10.7016) knots 0 0 0 1 2 3 3 3
  line L124 (11.9645, 10.7016) -> (11.8823, 10.7017)
  line L125 (11.8823, 10.7017) -> (11.884, 12.1186)
  spline S105 degree 2 poles (11.884, 12.1186) (11.8847, 12.6714) (12.0372, 13.1842) (12.4485, 13.5074) (12.7249, 13.5071) knots 0 0 0 1 2 3 3 3
  spline S106 degree 2 poles (12.7249, 13.5071) (13.0636, 13.5067) (13.2824, 13.2624) knots 0 0 0 1 1 1
  spline S107 degree 2 poles (13.2824, 13.2624) (13.4217, 13.1078) (13.4911, 12.8288) knots 0 0 0 1 1 1
  line L126 (13.4911, 12.8288) -> (14.5254, 13.5597)
  spline S108 degree 2 poles (14.5254, 13.5597) (14.7273, 13.7038) (14.7747, 13.766) knots 0 0 0 1 1 1
  spline S109 degree 2 poles (14.7747, 13.766) (14.8445, 13.8581) (14.8521, 13.9801) knots 0 0 0 1 1 1
  line L127 (14.8521, 13.9801) -> (14.9343, 13.98)
  line L128 (14.9343, 13.98) -> (14.9331, 13.0188)
  line L129 (14.9331, 13.0188) -> (13.5424, 12.0369)
  line L130 (13.5424, 12.0369) -> (13.5422, 11.8376)
  line L131 (12.048, 11.8395) -> (13.3828, 11.8378)
  line L132 (13.3828, 11.8378) -> (13.3829, 11.9648)
  spline S110 degree 2 poles (13.3829, 11.9648) (13.3833, 12.2786) (13.2692, 12.59) (12.9706, 12.7672) (12.729, 12.7675) knots 0 0 0 1 2 3 3 3
  spline S111 degree 2 poles (12.729, 12.7675) (12.3829, 12.7679) (12.0488, 12.4421) (12.0483, 12.081) knots 0 0 0 1 2 2 2
  line L133 (12.0483, 12.081) -> (12.048, 11.8395)
  point P0 (0, 0)
  constraints: 4 other
extrude "Extrusion20" cut sketch "Sketch26" against normal blind 7.62
body "Solid1"
